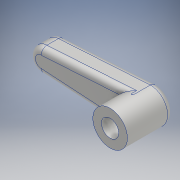
# Autodesk Inventor part: Reverse Gear Link Lever
Saved by Autodesk Inventor 2017 (Build 210142000, 142)
## iProperties
Created: 2018-11-07
Part Number: Reverse Gear Link Lever
Material: Aluminum 6061
Document SubType Name: Modeling
Designer: 623516
Density: 2.7 g/cm^3
Appearance: Aluminum - Flat
Author: 623516
Autodesk Inventor part; units mm, degrees
ref_plane "YZ Plane" through (0, 0, 0) normal (1, 0, 0) x (0, 1, 0)
ref_plane "XZ Plane" through (0, 0, 0) normal (0, 1, 0) x (-1, 0, 0)
ref_plane "XY Plane" through (0, 0, 0) normal (0, 0, 1) x (1, 0, 0)
sketch "Sketch1" plane through (0, 0, 0) normal (0, 1, 0) x (-1, 0, 0)
  circle A0 centre (0, 0) radius 3
  dimension "d0" = 6
  constraints: 1 centre point, 1 coincident
  measures "d0" diameter of A0
extrude "Extrusion1" add sketch "Sketch1" along normal blind 4
sketch "Sketch2" plane through (0, 4, 0) normal (0, 1, 0) x (1, 0, 0)
  line L0 (0, 0) -> (-16, 0) construction
  line L1 (-16, 0) -> (-16, 2) construction
  line L2 (-16, 0) -> (-16, -2) construction
  circle A0 centre (0, 0) radius 3 projected
  line L3 (0, -3) -> (-16, -2)
  line L4 (0, 3) -> (-16, 2)
  arc A1 (-16, 2) -> (-16, -2) centre (-16, 0) ccw
  dimension "d3" = 16
  dimension "d4" = 2
  dimension "d5" = 2
  dimension "d6" = 2
  constraints: 10 end point, 4 point on circle, 2 vertical, 1 centre point, 1 horizontal
  measures "d3" distance of L0.start L0.end
  measures "d4" distance of L0.end L1.end
  measures "d5" distance of L0.end L2.end
  measures "d6" radius of A1
extrude "Extrusion2" add sketch "Sketch2" along normal blind 4 contours A0 L3 L4 | A0 L3 A1 L4
fillet "Fillet1" radius 1 7 edges at (-8, 8, -2.5) (-18, 8, 0) (-8, 8, 2.5) (3, 8, 0) (-8.1868, 4, -2.4883) (-18, 4, 0) (-8.1868, 4, 2.4883)
sketch "Sketch3" plane through (0, 8, 0) normal (0, 1, 0) x (1, 0, 0)
  circle A0 centre (0, 0) radius 1.5
  dimension "d10" = 3
  constraints: 1 centre point, 1 coincident
  measures "d10" diameter of A0
extrude "Extrusion3" cut sketch "Sketch3" against normal blind 555
body "Solid1"
